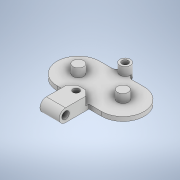
# Autodesk Inventor part: basedelapinza1
Saved by Autodesk Inventor 2021 (Build 250183000, 183)
## iProperties
Created: 2021-03-25
Part Number: basedelapinza1
Material: Genérico
Document SubType Name: Modeling
Designer: Arturo
Density: 1 g/cm^3
Appearance: Valor por defecto
Author: Arturo
Autodesk Inventor part; units mm, degrees
ref_plane "YZ Plane" through (0, 0, 0) normal (1, 0, 0) x (0, 1, 0)
ref_plane "XZ Plane" through (0, 0, 0) normal (0, 1, 0) x (-1, 0, 0)
ref_plane "XY Plane" through (0, 0, 0) normal (0, 0, 1) x (1, 0, 0)
sketch "Boceto1" plane through (0, 0, 0) normal (0, 1, 0) x (-1, 0, 0)
  circle A0 centre (0, 0) radius 2.5
  arc A1 (0, 10) -> (0, -10) centre (0, 0) ccw
  circle A2 centre (20.9, 0) radius 2.5
  arc A3 (20.9, -10) -> (20.9, 10) centre (20.9, 0) ccw
  line L0 (20.9, 10) -> (14.95, 10)
  line L1 (5.95, 10) -> (0, 10)
  line L2 (14.95, 10) -> (14.95, 24)
  line L3 (14.95, 24) -> (5.95, 24)
  line L4 (5.95, 24) -> (5.95, 10)
  line L5 (10.45, 9) -> (12.45, 9)
  line L6 (12.45, 9) -> (8.45, 9)
  circle A4 centre (10.45, 11.5) radius 1.5
  line L7 (12.45, 9) -> (14.95, 11.5)
  line L8 (8.45, 9) -> (5.95, 11.5)
  circle A5 centre (10.45, -11.5) radius 1.5
  arc A6 (8.0005, -12) -> (12.8995, -12) centre (10.45, -11.5) ccw
  line L9 (20.9, -10) -> (15.349, -10)
  line L10 (0, -10) -> (5.551, -10)
  arc A7 (8.0005, -12) -> (5.551, -10) centre (5.551, -12.5) ccw
  arc A8 (15.349, -10) -> (12.8995, -12) centre (15.349, -12.5) ccw
  circle A9 centre (10.45, -11.5) radius 2.5
  point P0 (8.45, -10)
  point P1 (12.45, -10)
  dimension "d10" = 5
  dimension "d11" = 20
  dimension "d13" = 5
  dimension "d14" = 20
  dimension "d19" = 9
  dimension "d20" = 14
  dimension "d25" = 3
  dimension "d27" = 3
  dimension "d28" = 5
  dimension "d29" = 2.5
  dimension "d30" = 5
  constraints: 22 end point, 12 point on circle, 10 centre point, 6 point on line, 6 tangent, 4 coincident, 2 horizontal, 1 equal radius, 1 parallel, 1 perpendicular
  measures "d10" diameter of A0
  measures "d11" diameter of A1
  measures "d13" diameter of A2
  measures "d14" diameter of A3
  measures "d19" distance of L3.end L2.end
  measures "d20" distance of L0.end L2.end
  measures "d25" diameter of A4
  measures "d27" diameter of A5
  measures "d28" diameter of A6
  measures "d29" radius of A7
  measures "d30" diameter of A9
extrude "Extrusión1" add sketch "Boceto1" along normal blind 6 contours A0 | L4 L3 L2 L7 L5 L6 L8 | A9 A6 | A2
extrude "Extrusión2" add sketch "Boceto1" along normal blind 2 contours L1 L4 L8 L6 L5 L7 L2 L0 A3 L9 A8 A9 A7 L10 A1
sketch "Boceto2" plane through (-5.95, 0, 24) normal (1, 0, 0) x (0, 0, -1)
  line L0 (0, 0) -> (14, 0) projected
  line L1 (14, 0) -> (14, 2) projected
  line L2 (12.5, 2) -> (14, 2) projected
  line L3 (12.5, 2) -> (12.5, 6) projected
  line L4 (0, 6) -> (12.5, 6) projected
  line L5 (0, 0) -> (0, 6) projected
  line L6 (0, 6) -> (12.5, 6) projected
  line L7 (0, 6) -> (0, 3)
  line L8 (0, 0) -> (0, 6) projected
  line L9 (0, 3) -> (3, 3)
  circle A0 centre (3, 3) radius 3
  circle A1 centre (3, 3) radius 1.75
  line L10 (0, 6) -> (3, 6)
  line L11 (0, 3) -> (0, 0)
  point P0 (24, 0)
  point P1 (3, 6)
  point P2 (3, 0)
  dimension "d37" = 6
  dimension "d35" = 3
  dimension "d36" = 3
  dimension "d38" = 3.5
  constraints: 8 end point, 2 coincident, 1 centre point, 1 collinear, 1 midpoint, 1 perpendicular, 1 point on line, 3 other
  measures "d35" distance of L4.start L7.end
  measures "d36" distance of L7.end L9.end
  measures "d38" diameter of A1
extrude "Extrusión3" cut sketch "Boceto2" against normal blind 9 contours L5 A0 L0 | A1 | L5 L4 A0
